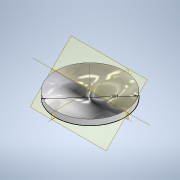
# Autodesk Inventor part: 1in_5mm_mir
Saved by Autodesk Inventor 2020 (Build 240168000, 168)
## iProperties
Created: 2019-05-24
Part Number: 1in_5mm_mir
Material: Generic
Document SubType Name: Modeling
Designer: Julian
Density: 1 g/cm^3
Appearance: Default
Author: Julian
Autodesk Inventor part; units mm, degrees
ref_plane "YZ Plane" through (0, 0, 0) normal (1, 0, 0) x (0, 1, 0)
ref_plane "XZ Plane" through (0, 0, 0) normal (0, 1, 0) x (-1, 0, 0)
ref_plane "XY Plane" through (0, 0, 0) normal (0, 0, 1) x (1, 0, 0)
sketch "Sketch1" plane through (0, 0, 0) normal (0, 1, 0) x (-1, 0, 0)
  circle A0 centre (0, 0) radius 12.5
  point P0 (0, -12.5)
  point P1 (-12.5, 0)
  dimension "d0" = 25
  constraints: 2 coincident, 2 point on circle, 1 centre point
  measures "d0" diameter of A0
extrude "Extrusion1" add sketch "Sketch1" along normal blind 2
ref_plane "Work Plane1" through (0, 0, 0) normal (1, 0, 0) x (0, 0, -1)
ref_plane "Work Plane2" through (12.5, 0, 0) normal (0, 0, -1) x (-1, 0, 0)
ref_plane "Work Plane4" through (0, 2, 0) normal (0, 0.7071, -0.7071) x (-1, 0, 0)
ref_plane "Work Plane5" through (0, 2, 0) normal (0, 0.7071, 0.7071) x (1, 0, 0)
body "Solid1"
